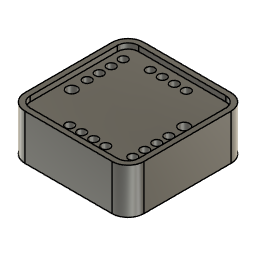
MouseBoxEIB16 v1 (Autodesk Fusion 360 design; units mm, degrees)
Autodesk Fusion 360 part; units mm, degrees
note: some values were not read from the file. Set by a fixed rule: which sketch regions a step uses.
sketch "Sketch2" plane through (0, 0, 0) normal (0, 0, 1) x (1, 0, 0)
  line L0 (4.1, 5.1) -> (-4.1, 5.1)
  line L1 (-5.1, 4.1) -> (-5.1, -4.1)
  line L2 (-4.1, -5.1) -> (4.1, -5.1)
  line L3 (5.1, -4.1) -> (5.1, 4.1)
  line L4 (5.1, 5.1) -> (-5.1, -5.1) construction
  line L5 (-5.1, 5.1) -> (5.1, -5.1) construction
  line L6 (4.1, 5.6) -> (-4.1, 5.6)
  line L7 (-5.6, 4.1) -> (-5.6, -4.1)
  line L8 (-4.1, -5.6) -> (4.1, -5.6)
  line L9 (5.6, -4.1) -> (5.6, 4.1)
  line L10 (5.6, 5.6) -> (-5.6, -5.6) construction
  line L11 (-5.6, 5.6) -> (5.6, -5.6) construction
  arc A0 (-4.1, 5.1) -> (-5.1, 4.1) centre (-4.1, 4.1) ccw
  arc A1 (5.1, 4.1) -> (4.1, 5.1) centre (4.1, 4.1) ccw
  arc A2 (4.1, -5.1) -> (5.1, -4.1) centre (4.1, -4.1) ccw
  arc A3 (-5.1, -4.1) -> (-4.1, -5.1) centre (-4.1, -4.1) ccw
  arc A4 (-5.6, -4.1) -> (-4.1, -5.6) centre (-4.1, -4.1) ccw
  arc A5 (4.1, -5.6) -> (5.6, -4.1) centre (4.1, -4.1) ccw
  arc A6 (5.6, 4.1) -> (4.1, 5.6) centre (4.1, 4.1) ccw
  arc A7 (-4.1, 5.6) -> (-5.6, 4.1) centre (-4.1, 4.1) ccw
  point P0 (-4.8071, 4.8071)
  point P1 (-5.1, 5.1)
  dimension "d84" = 10.2
  dimension "d85" = 10.2
  dimension "d86" = 11.2
  dimension "d87" = 11.2
  dimension "d88" = 1
  dimension "d89" = 1
  dimension "d90" = 1
  dimension "d91" = 1
  dimension "d92" = 1.5
  dimension "d93" = 1.5
  dimension "d94" = 1.5
  dimension "d95" = 1.5
  constraint horizontal L0
  constraint perpendicular L0 L1
  constraint parallel L0 L2
  constraint parallel L1 L3
  constraint coincident L4 origin
  constraint coincident L5 origin
  constraint horizontal L6
  constraint perpendicular L6 L7
  constraint parallel L6 L8
  constraint parallel L7 L9
  constraint coincident L10 origin
  constraint coincident L11 origin
  constraint coincident P1 L0
  constraint coincident P1 L1
  constraint tangent L0 A0
  constraint tangent L1 A0
  constraint midpoint A0 P0
  constraint coincident P1 L5.start
  constraint coincident L4.start L0
  constraint coincident L4.start L3
  constraint tangent L0 A1
  constraint tangent L3 A1
  constraint coincident L5.end L3
  constraint coincident L5.end L2
  constraint tangent L3 A2
  constraint tangent L2 A2
  constraint coincident L4.end L1
  constraint coincident L4.end L2
  constraint tangent L1 A3
  constraint tangent L2 A3
  constraint coincident L10.end L7
  constraint coincident L10.end L8
  constraint tangent L7 A4
  constraint tangent L8 A4
  constraint coincident L11.end L9
  constraint coincident L11.end L8
  constraint tangent L9 A5
  constraint tangent L8 A5
  constraint coincident L10.start L9
  constraint coincident L10.start L6
  constraint tangent L9 A6
  constraint tangent L6 A6
  constraint coincident L11.start L6
  constraint coincident L11.start L7
  constraint tangent L6 A7
  constraint tangent L7 A7
  measures "d84" distance of L4.end L5.end
  measures "d85" distance of P1 L4.end
  measures "d86" distance of L10.end L11.end
  measures "d87" distance of L11.start L10.end
  measures "d88" radius of A0
  measures "d89" radius of A1
  measures "d90" radius of A2
  measures "d91" radius of A3
  measures "d92" radius of A4
  measures "d93" radius of A5
  measures "d94" radius of A6
  measures "d95" radius of A7
extrude "Extrude1" add sketch "Sketch2" along normal blind 4.25
extrude "Extrude2" add sketch "Sketch2" along normal blind 3.75 contours L0 L1 L2 L3 A0 A1 A2 A3
sketch "Sketch4" plane through (0, 0, 3.75) normal (0, 0, 1) x (-1, 0, 0)
  line L0 (-5.05, 5) -> (5.05, 5)
  line L1 (5.05, 5) -> (5.05, -5)
  line L2 (5.05, -5) -> (-5.05, -5)
  line L3 (-5.05, -5) -> (-5.05, 5)
  line L4 (-5.05, 5) -> (5.05, -5) construction
  line L5 (5.05, 5) -> (-5.05, -5) construction
  line L6 (5.05, -4.1978) -> (4.2, -4.1978)
  line L7 (4.2, -4.1978) -> (4.2, -5)
  line L8 (4.2, -5) -> (4.2, -3.75)
  line L9 (4.2, -3.75) -> (4.2, -2.62)
  line L10 (4.2, -2.62) -> (4.2, -1.49)
  line L11 (4.2, -1.49) -> (4.2, -0.36)
  line L12 (4.2, -0.36) -> (4.2, 1.14)
  line L13 (4.2, 1.14) -> (5.05, 1.14)
  line L14 (5.05, 1.14) -> (4.15, 1.14)
  line L15 (3.2, -5) -> (3.2, -4.15)
  line L16 (3.2, -4.15) -> (5.05, -4.15)
  line L17 (5.05, -4.15) -> (2.05, -4.15)
  line L18 (2.05, -4.15) -> (0.92, -4.15)
  line L19 (0.92, -4.15) -> (-0.21, -4.15)
  line L20 (-0.21, -4.15) -> (-1.34, -4.15)
  line L21 (-3.0687, 5) -> (-3.0687, 4.15)
  line L22 (-3.0687, 4.15) -> (-5.05, 4.15)
  line L23 (-5.05, 4.15) -> (-2.05, 4.15)
  line L24 (-2.05, 4.15) -> (-0.92, 4.15)
  line L25 (-0.92, 4.15) -> (0.21, 4.15)
  line L26 (0.21, 4.15) -> (1.34, 4.15)
  line L27 (-5.05, 3.3083) -> (-4.2, 3.3083)
  line L28 (-4.2, 3.3083) -> (-4.2, 5)
  line L29 (-4.2, 5) -> (-4.2, 3.75)
  line L30 (-4.2, 3.75) -> (-4.2, 2.62)
  line L31 (-4.2, 2.62) -> (-4.2, 1.49)
  line L32 (-4.2, 1.49) -> (-4.2, 0.36)
  circle A0 centre (-1.34, -4.15) radius 0.4
  circle A1 centre (-0.21, -4.15) radius 0.4
  circle A2 centre (0.92, -4.15) radius 0.4
  circle A3 centre (2.05, -4.15) radius 0.4
  circle A4 centre (4.2, -3.75) radius 0.4
  circle A5 centre (4.2, -2.62) radius 0.4
  circle A6 centre (4.2, -1.49) radius 0.4
  circle A7 centre (4.2, -0.36) radius 0.4
  circle A8 centre (4.15, 1.14) radius 0.5
  circle A9 centre (1.34, 4.15) radius 0.4
  circle A10 centre (0.21, 4.15) radius 0.4
  circle A11 centre (-0.92, 4.15) radius 0.4
  circle A12 centre (-2.05, 4.15) radius 0.4
  circle A13 centre (-4.2, 3.75) radius 0.4
  circle A14 centre (-4.2, 2.62) radius 0.4
  circle A15 centre (-4.2, 1.49) radius 0.4
  circle A16 centre (-4.2, 0.36) radius 0.4
  line L33 (-4.2, 0.36) -> (-4.2, -1.14)
  line L34 (-4.2, -1.14) -> (-5.05, -1.14)
  line L35 (-5.05, -1.14) -> (-4.15, -1.14)
  circle A17 centre (-4.15, -1.14) radius 0.5
  point P0 (4.15, 1.14)
  point P1 (4.2, -0.36)
  point P2 (4.2, -1.49)
  point P3 (4.2, -2.62)
  point P4 (4.2, -3.75)
  point P5 (2.05, -4.15)
  point P6 (0.92, -4.15)
  point P7 (-0.21, -4.15)
  point P8 (1.34, 4.15)
  point P9 (-2.05, 4.15)
  point P10 (-0.92, 4.15)
  point P11 (0.21, 4.15)
  point P12 (-4.2, 3.75)
  point P13 (-4.2, 2.62)
  point P14 (-4.2, 1.49)
  point P15 (-4.2, 0.36)
  dimension "d140" = 10.1
  dimension "d141" = 10
  dimension "d142" = 0.85
  dimension "d143" = 1.25
  dimension "d144" = 1.13
  dimension "d145" = 1.13
  dimension "d146" = 1.13
  dimension "d147" = 1.5
  dimension "d148" = 0.9
  dimension "d149" = 0.85
  dimension "d150" = 3
  dimension "d151" = 1.13
  dimension "d152" = 1.13
  dimension "d153" = 1.13
  dimension "d154" = 0.85
  dimension "d155" = 3
  dimension "d156" = 1.13
  dimension "d157" = 1.13
  dimension "d158" = 1.13
  dimension "d160" = 0.85
  dimension "d161" = 1.25
  dimension "d162" = 1.13
  dimension "d163" = 1.13
  dimension "d164" = 1.13
  dimension "d165" = 0.8
  dimension "d166" = 0.8
  dimension "d167" = 0.8
  dimension "d168" = 0.8
  dimension "d169" = 0.8
  dimension "d170" = 0.8
  dimension "d171" = 0.8
  dimension "d172" = 0.8
  dimension "d173" = 1
  dimension "d174" = 0.8
  dimension "d175" = 0.8
  dimension "d176" = 0.8
  dimension "d177" = 0.8
  dimension "d178" = 0.8
  dimension "d179" = 0.8
  dimension "d180" = 0.8
  dimension "d181" = 0.8
  dimension "d182" = 1.5
  dimension "d183" = 0.9
  dimension "d184" = 1
  constraint horizontal L0
  constraint perpendicular L0 L1
  constraint parallel L0 L2
  constraint parallel L1 L3
  constraint coincident L4 origin
  constraint coincident L5 origin
  constraint coincident L1 L6.start
  constraint perpendicular L1 L6
  constraint coincident L2 L7.end
  constraint perpendicular L2 L7
  constraint perpendicular L2 L8
  constraint parallel L8 L9
  constraint parallel L9 L10
  constraint parallel L10 L11
  constraint parallel L11 L12
  constraint coincident L1 L13.end
  constraint perpendicular L1 L13
  constraint perpendicular L12 L14
  constraint coincident P0 L14.end
  constraint coincident P1 L11.end
  constraint coincident P2 L10.end
  constraint coincident P3 L9.end
  constraint coincident P4 L8.end
  constraint coincident L2 L15.start
  constraint perpendicular L2 L15
  constraint coincident L1 L16.end
  constraint perpendicular L1 L16
  constraint perpendicular L15 L17
  constraint perpendicular L15 L18
  constraint parallel L18 L19
  constraint parallel L19 L20
  constraint coincident P5 L17.end
  constraint coincident P6 L18.end
  constraint coincident P7 L19.end
  constraint coincident L0 L21.start
  constraint perpendicular L0 L21
  constraint coincident L3 L22.end
  constraint perpendicular L3 L22
  constraint perpendicular L21 L23
  constraint perpendicular L21 L24
  constraint perpendicular L21 L25
  constraint parallel L25 L26
  constraint coincident P8 L26.end
  constraint coincident P9 L23.end
  constraint coincident P10 L24.end
  constraint coincident P11 L25.end
  constraint coincident L3 L27.start
  constraint perpendicular L3 L27
  constraint coincident L0 L28.end
  constraint perpendicular L0 L28
  constraint perpendicular L23 L29
  constraint parallel L28 L30
  constraint parallel L30 L31
  constraint parallel L31 L32
  constraint coincident P12 L29.end
  constraint coincident P13 L30.end
  constraint coincident P14 L31.end
  constraint coincident P15 L32.end
  constraint coincident L20.end A0.centre
  constraint parallel L32 L33
  constraint coincident L3 L34.end
  constraint perpendicular L3 L34
  constraint perpendicular L3 L35
  constraint coincident L35.end A17.centre
  measures "d140" distance of L1.end L2.end
  measures "d141" distance of L0.end L1.end
  measures "d142" distance of L6.start L6.end
  measures "d143" distance of L7.end P4
  measures "d144" distance of P4 P3
  measures "d145" distance of P3 P2
  measures "d146" distance of P2 P1
  measures "d147" distance of P1 L12.end
  measures "d148" distance of L13.end P0
  measures "d149" distance of L15.start L15.end
  measures "d150" distance of L16.end P5
  measures "d151" distance of P5 P6
  measures "d152" distance of P6 P7
  measures "d153" distance of P7 L20.end
  measures "d154" distance of L21.start L21.end
  measures "d155" distance of L22.end P9
  measures "d156" distance of P9 P10
  measures "d157" distance of P10 P11
  measures "d158" distance of P11 P8
  measures "d160" distance of L27.start L27.end
  measures "d161" distance of L28.end P12
  measures "d162" distance of P12 P13
  measures "d163" distance of P13 P14
  measures "d164" distance of P14 P15
  measures "d165" diameter of A0
  measures "d166" diameter of A1
  measures "d167" diameter of A2
  measures "d168" diameter of A3
  measures "d169" diameter of A4
  measures "d170" diameter of A5
  measures "d171" diameter of A6
  measures "d172" diameter of A7
  measures "d173" diameter of A8
  measures "d174" diameter of A9
  measures "d175" diameter of A10
  measures "d176" diameter of A11
  measures "d177" diameter of A12
  measures "d178" diameter of A13
  measures "d179" diameter of A14
  measures "d180" diameter of A15
  measures "d181" diameter of A16
  measures "d182" distance of P15 L33.end
  measures "d183" distance of L34.end L35.end
  measures "d184" diameter of A17
extrude "Extrude6" cut sketch "Sketch4" against normal blind 1 contours L28 L29 L30 A13 | L28 L29 L30 A13 | L33 L34 L35 A17 | L33 L34 L35 A17 | L30 L31 A14 | L30 L31 A14 | L12 L13 L14 A8 | L12 L13 L14 A8 | L8 L9 A4 | L8 L9 A4 | L32 A16 L33 | L32 A16 L33 | L31 L32 A15 | L31 L32 A15 | L11 L12 A7 | L11 L12 A7 | L9 L10 A5 | L9 L10 A5 | L10 L11 A6 | L10 L11 A6 | L17 L18 A3 | L17 L18 A3 | L18 L19 A2 | L18 L19 A2 | L19 L20 A1 | L19 L20 A1 | L23 L24 A12 | L23 L24 A12 | L24 L25 A11 | L24 L25 A11 | L25 L26 A10 | L25 L26 A10 | A0 | A9
